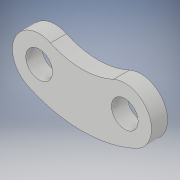
# Autodesk Inventor part: linkageC_mini
Saved by Autodesk Inventor 2017 (Build 210142000, 142)
## iProperties
Created: 2016-08-20
Part Number: linkageC_mini
Material: Generic
Document SubType Name: Modeling
Designer: Nic
Density: 1 g/cm^3
Appearance: Default
Author: Nic
Autodesk Inventor part; units mm, degrees
ref_plane "YZ Plane" through (0, 0, 0) normal (1, 0, 0) x (0, 1, 0)
ref_plane "XZ Plane" through (0, 0, 0) normal (0, 1, 0) x (-1, 0, 0)
ref_plane "XY Plane" through (0, 0, 0) normal (0, 0, 1) x (1, 0, 0)
sketch "Sketch1" plane through (0, 0, 0) normal (0, 0, 1) x (1, 0, 0)
  circle A0 centre (0, 0) radius 1.25
  line L0 (0, 0) -> (8, 0) construction
  circle A1 centre (8, 0) radius 1.25
  arc A2 (1.0526, 2.2676) -> (-1.0526, -2.2676) centre (0, 0) ccw
  arc A3 (9.0526, -2.2676) -> (6.9474, 2.2676) centre (8, 0) ccw
  arc A4 (-1.0526, -2.2676) -> (9.0526, -2.2676) centre (4, 8.6168) ccw
  arc A5 (1.0526, 2.2676) -> (4, 1.6168) centre (4, 8.6168) ccw
  arc A6 (4, 1.6168) -> (6.9474, 2.2676) centre (4, 8.6168) ccw
  dimension "d0" = 2.5
  dimension "d1" = 8
  dimension "d8" = 5
  dimension "d20" = 12
  constraints: 10 point on circle, 7 centre point, 5 coincident, 4 tangent, 3 equal radius, 2 end point, 1 concentric, 1 horizontal
  measures "d0" diameter of A0
  measures "d1" distance of L0.start L0.end
  measures "d8" diameter of A2
  measures "d20" radius of A4
extrude "Extrusion1" add sketch "Sketch1" along normal blind 1.5
body "Solid1"
